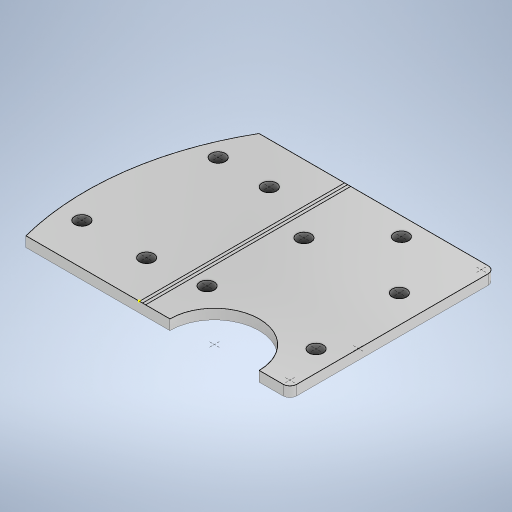
# Autodesk Inventor part: axis_2_bottom_L_frame(top)
Saved by Autodesk Inventor 2024.2 (Build 282272000, 272)
## iProperties
Created: 2023-12-25
Part Number: axis_2_bottom_L_frame(top)
Material: Aluminum 6061-AHC
Document SubType Name: Modeling
Designer: chanh
Density: 2.7 g/cm^3
Appearance: Aluminum - Dark
Author: chanh
Autodesk Inventor part; units mm, degrees
ref_plane "YZ Plane" through (0, 0, 0) normal (1, 0, 0) x (0, 1, 0)
ref_plane "XZ Plane" through (0, 0, 0) normal (0, 1, 0) x (-1, 0, 0)
ref_plane "XY Plane" through (0, 0, 0) normal (0, 0, 1) x (1, 0, 0)
sketch "Sketch1" plane through (0, 0, 0) normal (0, 1, 0) x (-1, 0, 0)
  line L0 (-0.4496, -30.1) -> (-0.4496, 0)
  circle A0 centre (14.5, -6.05) radius 1.05
  circle A1 centre (12.5, -24.05) radius 1.05
  circle A2 centre (5, -24.05) radius 1.05
  circle A3 centre (5, -6.05) radius 1.05
  circle A4 centre (-19.0193, -6.9) radius 1.05
  circle A5 centre (-18.0193, -20.12) radius 1.05
  circle A6 centre (-11.0193, -27.42) radius 1.05
  circle A7 centre (-4.0193, -20.12) radius 1.05
  circle A8 centre (-3.0193, -6.9) radius 1.05
  arc A9 (-21.0893, 0) -> (-22.0893, -1) centre (-21.0893, -1) ccw
  line L1 (-22.0893, -29.1) -> (-22.0893, -1)
  arc A10 (-22.0893, -29.1) -> (-21.0893, -30.1) centre (-21.0893, -29.1) ccw
  arc A11 (12.5521, -30.1) -> (16.6569, 0) centre (-22.06, -10.05) ccw
  line L2 (-4.4693, 0) -> (16.6569, 0)
  line L3 (12.5521, -30.1) -> (-21.0893, -30.1)
  arc A12 (-17.5693, 0) -> (-4.4693, 0) centre (-11.0193, 0) ccw
  line L4 (-21.0893, 0) -> (-17.5693, 0)
  line L5 (-0.8993, -30.1) -> (-0.8993, 0)
  line L6 (0, 0) -> (0, -30.1)
  constraints: 14 end point, 13 centre point, 8 point on circle, 6 point on line, 4 vertical, 3 horizontal, 41 other
extrude "Extrusion1" add sketch "Sketch1" against normal blind 1.5
body "Solid1"
